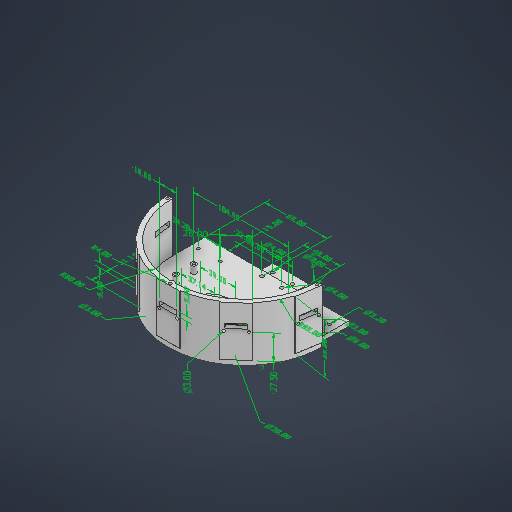
# Autodesk Inventor part: Mitad_1
Saved by Autodesk Inventor 2026.2 (Build 302298000, 298)
## iProperties
Created: 2025-10-28
Part Number: Mitad_1
Material: Genérico
Document SubType Name: Modeling
Designer: 100094631
Density: 1 g/cm^3
Appearance: Valor por defecto
Author: 100094631
## iProperties of the stored document Mitad_1_3DPrint.ipt
Created: 2026-02-23
Part Number: Mitad_1_3DPrint
Material: Genérico
Document SubType Name: Modeling
Designer: yahir
Density: 1 g/cm^3
Appearance: Valor por defecto
Author: yahir
Autodesk Inventor part; units mm, degrees
ref_plane "YZ Plane" through (0, 0, 0) normal (1, 0, 0) x (0, 1, 0)
ref_plane "XZ Plane" through (0, 0, 0) normal (0, 1, 0) x (-1, 0, 0)
ref_plane "XY Plane" through (0, 0, 0) normal (0, 0, 1) x (1, 0, 0)
sketch "Boceto2" plane through (0, 0, 0) normal (0, 1, 0) x (-1, 0, 0)
  arc A0 (85, 0) -> (-85, 0) centre (0, 0) ccw
  line L0 (85, 0) -> (80, 0)
  line L1 (-80, 0) -> (-85, 0)
  line L2 (80, 0) -> (80, -36)
  line L3 (-80, 0) -> (-80, -36)
  line L4 (-80, -36) -> (80, -36)
  point P0 (0, 0)
  point P1 (0, 85)
  dimension "d228" = 85
  dimension "d229" = 5
  dimension "d461" = 36
  dimension "d462" = 36
  constraints: 10 end point, 3 point on circle, 2 vertical, 1 centre point, 1 horizontal, 1 point on line
  measures "d228" distance of point (0, 0) L1.end
  measures "d229" distance of L0.start L0.end
  measures "d461" distance of L0.end L2.end
  measures "d462" distance of L1.start L3.end
extrude "Extrusión1" add sketch "Boceto2" along normal blind 5
sketch "Boceto6" plane through (0, 5, 0) normal (0, 1, 0) x (1, 0, 0)
  circle A0 centre (48.25, 21) radius 1.6
  circle A1 centre (72.45, 21) radius 1.6
  circle A2 centre (-72.45, 21) radius 1.6
  line L0 (80, 36) -> (-80, 36) projected
  line L1 (80, 36) -> (80, 21)
  line L2 (80, 0) -> (80, 36) projected
  line L3 (80, 21) -> (72.45, 21)
  line L4 (-80, 36) -> (-80, 0) projected
  line L5 (-80, 36) -> (-80, 21)
  line L6 (-80, 21) -> (-72.45, 21)
  line L7 (72.45, 21) -> (48.25, 21)
  line L8 (-72.45, 21) -> (-48.25, 21)
  circle A3 centre (-48.25, 21) radius 1.6
  dimension "d59" = 3.2
  dimension "d60" = 3.2
  dimension "d63" = 3.2
  dimension "d468" = 15
  dimension "d469" = 7.55
  dimension "d471" = 15
  dimension "d472" = 7.55
  dimension "d502" = 24.2
  dimension "d503" = 24.2
  dimension "d504" = 3.2
  constraints: 12 end point, 4 centre point, 3 point on line, 2 perpendicular, 1 coincident, 1 horizontal
  measures "d59" diameter of A0
  measures "d60" diameter of A1
  measures "d63" diameter of A2
  measures "d468" distance of L0.start L1.end
  measures "d469" distance of L1.end L3.end
  measures "d471" distance of L0.end L5.end
  measures "d472" distance of L5.end L6.end
  measures "d502" distance of L3.end L7.end
  measures "d503" distance of L6.end L8.end
  measures "d504" diameter of A3
extrude "Extrusión4" cut sketch "Boceto6" against normal blind 5
sketch "Boceto7" plane through (0, 5, 0) normal (0, 1, 0) x (1, 0, 0)
  line L0 (0, 0) -> (0, -85)
  line L1 (0, 0) -> (55.2031, -64.6345)
  line L2 (0, 0) -> (83.9535, -13.2969)
  arc A0 (-80, 0) -> (80, 0) centre (0, 0) ccw
  line L3 (-85, 0) -> (-80, 0)
  line L4 (80, 0) -> (85, 0)
  line L5 (0, -85) -> (13, -85)
  arc A1 (-85, 0) -> (85, 0) centre (0, 0) ccw projected
  line L6 (0, -85) -> (-13, -85)
  line L7 (-13, -85) -> (-13, -84)
  line L8 (13, -85) -> (13, -84)
  line L9 (0, 0) -> (-55.2031, -64.6345)
  line L10 (0, 0) -> (85, 0) construction
  line L11 (0, 0) -> (85, 0) construction
  line L12 (0, 0) -> (-83.9535, -13.2969)
  line L13 (0, 0) -> (90.9011, 0) construction
  line L14 (0, 0) -> (55.2031, -64.6345)
  line L15 (55.2031, -64.6345) -> (65.0884, -56.1917)
  line L16 (55.2031, -64.6345) -> (45.3178, -73.0773)
  line L17 (45.3178, -73.0773) -> (44.6684, -72.3169)
  line L18 (65.0884, -56.1917) -> (64.4389, -55.4313)
  line L19 (0, 0) -> (83.9535, -13.2969)
  line L20 (83.9535, -13.2969) -> (85.9872, -0.457)
  line L21 (83.9535, -13.2969) -> (81.9199, -26.1369)
  line L22 (81.9199, -26.1369) -> (80.9322, -25.9804)
  line L23 (85.9872, -0.457) -> (84.9995, -0.3005)
  line L24 (0, 0) -> (-55.2031, -64.6345)
  line L25 (-55.2031, -64.6345) -> (-45.3178, -73.0773)
  line L26 (-55.2031, -64.6345) -> (-65.0884, -56.1917)
  line L27 (-65.0884, -56.1917) -> (-64.4389, -55.4313)
  line L28 (-45.3178, -73.0773) -> (-44.6684, -72.3169)
  line L29 (0, 0) -> (-83.9535, -13.2969)
  line L30 (-83.9535, -13.2969) -> (-81.9199, -26.1369)
  line L31 (-83.9535, -13.2969) -> (-85.9872, -0.457)
  line L32 (-85.9872, -0.457) -> (-84.9995, -0.3005)
  line L33 (-81.9199, -26.1369) -> (-80.9322, -25.9804)
  arc A2 (-85, 0) -> (-84.9995, -0.3005) centre (0, 0) ccw
  arc A3 (-80.9322, -25.9804) -> (-64.4389, -55.4313) centre (0, 0) ccw
  arc A4 (-44.6684, -72.3169) -> (-13, -84) centre (0, 0) ccw
  arc A5 (13, -84) -> (44.6684, -72.3169) centre (0, 0) ccw
  arc A6 (64.4389, -55.4313) -> (80.9322, -25.9804) centre (0, 0) ccw
  arc A7 (84.9995, -0.3005) -> (85, 0) centre (0, 0) ccw
  point P0 (0, 0)
  point P1 (-80, 0)
  dimension "d234" = 40.5
  dimension "d235" = 81
  dimension "d237" = 13
  dimension "d238" = 13
  dimension "d241" = 171
  dimension "d242" = 13
  dimension "d243" = 13
  dimension "d244" = 13
  dimension "d245" = 13
  dimension "d246" = 13
  dimension "d247" = 13
  dimension "d248" = 13
  dimension "d249" = 13
  constraints: 68 end point, 17 point on circle, 7 centre point, 7 horizontal, 5 perpendicular, 3 tangent, 2 vertical, 1 coincident, 1 equal length
  measures "d234" angle of L1 L0
  measures "d235" angle of L2 L0
  measures "d237" distance of L0.end L5.end
  measures "d238" distance of L0.end L6.end
  measures "d241" angle of L12 L13
  measures "d242" distance of L15.start L15.end
  measures "d243" distance of L15.start L16.end
  measures "d244" distance of L21.start L20.end
  measures "d245" distance of L21.start L21.end
  measures "d246" distance of L24.end L25.end
  measures "d247" distance of L24.end L27.start
  measures "d248" distance of L29.end L33.start
  measures "d249" distance of L29.end L31.end
extrude "Extrusión5" add sketch "Boceto7" along normal blind 55 contours A0 L1 A1 L0 | L0 A1 L9 A0 | A0 L2 A1 L1 | A0 L4 A1 L2 | L9 A1 L12 A0 | L12 A1 L3 A0 | A1 L8 L5 | L6 L7 A1 | L16 L17 A1 | A1 L18 L15 | L21 L22 A1 | A1 L23 L20 | L26 L27 A1 | A1 L28 L25 | L31 L32 A1 | A1 L33 L30
sketch "Boceto22" plane through (0, 5, 0) normal (0, 1, 0) x (1, 0, 0)
  ellipse E0 centre (0, -30) end of major axis (0, -12.5) minor radius 25
  line L0 (0, -30) -> (-0.3651, -30)
  line L1 (-80, 36) -> (0, 36)
  line L2 (80, 36) -> (-80, 36) projected
  line L3 (-80, 36) -> (-80, 0) projected
  line L4 (-80, 36) -> (0, 36)
  line L5 (0, 36) -> (0, -30)
  point P0 (0, 0)
  dimension "d473" = 80
  constraints: 8 end point, 1 collinear, 1 horizontal, 1 midpoint, 1 vertical, 2 other
  measures "d473" distance of L1.start L1.end
extrude "Extrusión15" add sketch "Boceto22" along normal blind 3.3
sketch "Boceto25" plane through (0, 60, 0) normal (0, 1, 0) x (1, 0, 0)
  circle A0 centre (82.75, -3) radius 1.5
  circle A1 centre (-82.75, -3) radius 1.5
  circle A2 centre (0, -82.5) radius 1.5
  line L0 (0, -85) -> (0, -82.5)
  line L1 (82.75, 0) -> (82.75, -3)
  line L2 (-82.75, 0) -> (-82.75, -3)
  line L3 (85, 0) -> (80, 0) projected
  line L4 (80, 0) -> (82.75, 0)
  line L5 (-80, 0) -> (-82.75, 0)
  line L6 (-80, 0) -> (-85, 0) projected
  arc A3 (4, -82.5) -> (-4, -82.5) centre (0, -82.5) ccw
  line L7 (0, -82.5) -> (-4, -82.5)
  line L8 (0, -82.5) -> (4, -82.5)
  point P0 (0, 0)
  point P1 (-1.5, -82.5)
  point P2 (1.5, -82.5)
  dimension "d200" = 3
  dimension "d203" = 3
  dimension "d205" = 3
  dimension "d264" = 3
  dimension "d267" = 3
  dimension "d423" = 2.75
  dimension "d424" = 2.75
  dimension "d460" = 2.5
  constraints: 14 end point, 4 centre point, 3 point on line, 2 point on circle, 1 coincident, 1 horizontal, 1 vertical
  measures "d200" diameter of A0
  measures "d203" diameter of A1
  measures "d205" diameter of A2
  measures "d264" distance of L1.start L1.end
  measures "d267" distance of L2.start L2.end
  measures "d423" distance of L3.end L4.end
  measures "d424" distance of L5.start L5.end
  measures "d460" distance of L0.start L0.end
extrude "Extrusión17" cut sketch "Boceto25" against normal blind 5 contours A0 | A1 | L8 L7 A2 | A2 L0 L8 | L7 L0 A2
sketch "Boceto27" plane through (0, 8.3, 0) normal (0, 1, 0) x (1, 0, 0)
  ellipse E0 centre (0, -30) end of major axis (-25, -30) minor radius 17.5 projected
  circle A0 centre (0, -30) radius 15
  line L0 (0, -30) -> (-19.5, -30)
  line L1 (0, -30) -> (19.5, -30)
  circle A1 centre (19.5, -30) radius 2
  circle A2 centre (-19.5, -30) radius 2
  point P0 (0, 0)
  dimension "d252" = 30
  dimension "d253" = 19.5
  dimension "d254" = 19.5
  dimension "d255" = 4
  dimension "d256" = 4
  constraints: 4 end point, 3 centre point, 3 coincident, 2 horizontal, 1 other
  measures "d252" diameter of A0
  measures "d253" distance of L0.start L0.end
  measures "d254" distance of L0.start L1.end
  measures "d255" diameter of A1
  measures "d256" diameter of A2
extrude "Extrusión19" cut sketch "Boceto27" against normal blind 15 contours L1 L0 A0 | A2 | A0 L0 L1 | A1
sketch "Boceto31" plane through (-13, 5, 85) normal (0, 0, 1) x (1, 0, 0)
  line L0 (26, 0) -> (26, 55) projected
  line L1 (26, 0) -> (13, 0)
  line L2 (-12, 0) -> (38, 0) projected
  line L3 (13, 0) -> (13, 27.5)
  line L4 (13, 27.5) -> (23, 27.5)
  line L5 (13, 27.5) -> (3, 27.5)
  circle A0 centre (3, 27.5) radius 1.5
  circle A1 centre (23, 27.5) radius 1.5
  point P0 (13, -5)
  dimension "d282" = 13
  dimension "d283" = 27.5
  dimension "d285" = 10
  dimension "d286" = 3
  dimension "d287" = 3
  constraints: 8 end point, 2 centre point, 2 coincident, 2 horizontal, 1 midpoint, 1 perpendicular
  measures "d282" distance of L0.start L1.end
  measures "d283" distance of L1.end L3.end
  measures "d285" distance of L3.end L5.end
  measures "d286" diameter of A0
  measures "d287" diameter of A1
extrude "Extrusión23" cut sketch "Boceto31" against normal blind 3
sketch "Boceto32" plane through (65.0884, 5, 56.1917) normal (0.6494, 0, 0.7604) x (0.7604, 0, -0.6494)
  line L0 (-26, 0) -> (-26, 55) projected
  line L1 (-26, 0) -> (-13, 0)
  line L2 (-54.632, 0) -> (-10.3349, 0) projected
  line L3 (-13, 0) -> (-13, 27.5)
  line L4 (-13, 27.5) -> (-3, 27.5)
  line L5 (-13, 27.5) -> (-23, 27.5)
  circle A0 centre (-23, 27.5) radius 1.5
  circle A1 centre (-3, 27.5) radius 1.5
  point P0 (-13, -5)
  dimension "d290" = 13
  dimension "d291" = 27.5
  dimension "d292" = 10
  dimension "d293" = 10
  dimension "d294" = 3
  dimension "d295" = 3
  constraints: 8 end point, 2 centre point, 2 coincident, 2 horizontal, 1 perpendicular, 1 point on line
  measures "d290" distance of L0.start L1.end
  measures "d291" distance of L1.end L3.end
  measures "d292" distance of L3.end L4.end
  measures "d293" distance of L3.end L5.end
  measures "d294" diameter of A0
  measures "d295" diameter of A1
extrude "Extrusión24" cut sketch "Boceto32" against normal blind 3
sketch "Boceto33" plane through (85.9872, 5, 0.457) normal (0.9877, 0, 0.1564) x (0.1564, 0, -0.9877)
  line L0 (0.0086, 0) -> (-12.9914, 0)
  line L1 (-0.4852, 0) -> (-93, 0) projected
  line L2 (-12.9914, 0) -> (-12.9914, 27.5)
  line L3 (-12.9914, 27.5) -> (-2.9914, 27.5)
  line L4 (-12.9914, 27.5) -> (-22.9914, 27.5)
  circle A0 centre (-22.9914, 27.5) radius 1.5
  circle A1 centre (-2.9914, 27.5) radius 1.5
  point P0 (-13, -5)
  point P1 (-25.5148, 0)
  dimension "d298" = 13
  dimension "d299" = 27.5
  dimension "d300" = 10
  dimension "d301" = 10
  dimension "d302" = 3
  dimension "d303" = 3
  constraints: 8 end point, 2 centre point, 2 coincident, 2 perpendicular, 1 horizontal, 1 point on line
  measures "d298" distance of L0.start L0.end
  measures "d299" distance of L0.end L2.end
  measures "d300" distance of L2.end L3.end
  measures "d301" distance of L2.end L4.end
  measures "d302" diameter of A0
  measures "d303" diameter of A1
extrude "Extrusión25" cut sketch "Boceto33" against normal blind 3
sketch "Boceto34" plane through (-45.3178, 5, 73.0773) normal (-0.6494, 0, 0.7604) x (0.7604, 0, 0.6494)
  line L0 (67, 0) -> (-73.8325, 0) projected
  line L1 (-26.0047, 0) -> (-13.0047, 0)
  line L2 (-13.0047, 0) -> (-13.0047, 27.5)
  line L3 (-15.6651, 0) -> (28.632, 0) projected
  line L4 (-13.0047, 0) -> (14.4953, 0) construction
  line L5 (-13.0047, 27.5) -> (-3.0047, 27.5)
  line L6 (-13.0047, 27.5) -> (-23.0047, 27.5)
  circle A0 centre (-23.0047, 27.5) radius 1.5
  circle A1 centre (-3.0047, 27.5) radius 1.5
  point P0 (-13, -5)
  point P1 (47.8325, 0)
  dimension "d306" = 13
  dimension "d307" = 27.5
  dimension "d308" = 90
  dimension "d309" = 10
  dimension "d310" = 10
  dimension "d311" = 3
  dimension "d312" = 3
  constraints: 10 end point, 3 horizontal, 2 centre point, 2 coincident, 2 perpendicular, 2 point on line
  measures "d306" distance of L1.start L1.end
  measures "d307" distance of L1.end L2.end
  measures "d308" angle of L4 L2
  measures "d309" distance of L2.end L5.end
  measures "d310" distance of L2.end L6.end
  measures "d311" diameter of A0
  measures "d312" diameter of A1
extrude "Extrusión26" cut sketch "Boceto34" against normal blind 3
sketch "Boceto35" plane through (-81.9199, 5, 26.1369) normal (-0.9877, 0, 0.1564) x (0.1564, 0, 0.9877)
  line L0 (-27.7935, 0) -> (-24.5935, 0) projected
  line L1 (-25.9863, 0) -> (-12.9863, 0)
  line L2 (-12.9863, 0) -> (-12.9863, 27.5)
  line L3 (-12.9863, 27.5) -> (-2.9863, 27.5)
  line L4 (-12.9863, 27.5) -> (-22.9863, 27.5)
  circle A0 centre (-22.9863, 27.5) radius 1.5
  circle A1 centre (-2.9863, 27.5) radius 1.5
  point P0 (-13, -5)
  dimension "d315" = 13
  dimension "d316" = 27.5
  dimension "d317" = 10
  dimension "d318" = 10
  dimension "d319" = 3
  dimension "d320" = 3
  constraints: 8 end point, 2 centre point, 2 coincident, 2 perpendicular, 1 collinear, 1 horizontal, 1 point on line
  measures "d315" distance of L1.start L1.end
  measures "d316" distance of L1.end L2.end
  measures "d317" distance of L2.end L3.end
  measures "d318" distance of L2.end L4.end
  measures "d319" diameter of A0
  measures "d320" diameter of A1
extrude "Extrusión27" cut sketch "Boceto35" against normal blind 3
sketch "Boceto36" plane through (-13, 5, 85) normal (0, 0, 1) x (1, 0, 0)
  circle A0 centre (3, 27.5) radius 1.5 projected
  line L0 (3, 27.5) -> (13, 27.5)
  line L1 (13, 27.5) -> (13, 32.5)
  line L2 (4, 32.5) -> (4, 35)
  line L3 (4, 35) -> (22, 35)
  line L4 (22, 35) -> (22, 30)
  line L5 (22, 30) -> (4, 30)
  line L6 (4, 30) -> (4, 32.5)
  point P0 (13, -5)
  dimension "d336" = 10
  dimension "d337" = 5
  dimension "d340" = 2.5
  dimension "d358" = 18
  dimension "d359" = 5
  dimension "d360" = 18
  constraints: 14 end point, 2 horizontal, 2 perpendicular, 2 vertical
  measures "d336" distance of L0.start L0.end
  measures "d337" distance of L0.end L1.end
  measures "d340" distance of L2.start L2.end
  measures "d358" distance of L2.end L3.end
  measures "d359" distance of L3.end L4.end
  measures "d360" distance of L4.end L5.end
extrude "Extrusión28" cut sketch "Boceto36" against normal blind 6 contours L5 L6 L2 L3 L4
sketch "Boceto37" plane through (65.0884, 5, 56.1917) normal (0.6494, 0, 0.7604) x (0.7604, 0, -0.6494)
  circle A0 centre (-23, 27.5) radius 1.5 projected
  line L0 (-23, 27.5) -> (-13, 27.5)
  line L1 (-13, 27.5) -> (-13, 32.5)
  line L2 (-13, 32.5) -> (-4, 32.5)
  line L3 (-4, 32.5) -> (-4, 30)
  line L4 (-4, 30) -> (-22, 30)
  line L5 (-22, 30) -> (-22, 35)
  line L6 (-22, 35) -> (-4, 35)
  line L7 (-4, 35) -> (-4, 32.5)
  point P0 (-13, -5)
  dimension "d348" = 10
  dimension "d349" = 5
  dimension "d350" = 9
  dimension "d351" = 2.5
  dimension "d352" = 18
  dimension "d354" = 5
  dimension "d355" = 18
  constraints: 16 end point, 3 vertical, 2 horizontal, 2 perpendicular
  measures "d348" distance of L0.start L0.end
  measures "d349" distance of L0.end L1.end
  measures "d350" distance of L1.end L2.end
  measures "d351" distance of L2.end L3.end
  measures "d352" distance of L3.end L4.end
  measures "d354" distance of L4.end L5.end
  measures "d355" distance of L5.end L6.end
extrude "Extrusión29" cut sketch "Boceto37" against normal blind 6 contours L4 L5 L6 L7 L2 L1 | L1 L2 L3 L4
sketch "Boceto38" plane through (85.9872, 5, 0.457) normal (0.9877, 0, 0.1564) x (0.1564, 0, -0.9877)
  circle A0 centre (-22.9914, 27.5) radius 1.5 projected
  line L0 (-22.9914, 27.5) -> (-12.9914, 27.5)
  line L1 (-12.9914, 27.5) -> (-12.9914, 32.5)
  line L2 (-12.9914, 32.5) -> (-3.9914, 32.5)
  line L3 (-3.9914, 35) -> (-21.9914, 35)
  line L4 (-21.9914, 35) -> (-21.9914, 30)
  line L5 (-21.9914, 30) -> (-3.9914, 30)
  line L6 (-3.9914, 30) -> (-3.9914, 35)
  point P0 (-13, -5)
  dimension "d361" = 10
  dimension "d362" = 5
  dimension "d364" = 2.5
  dimension "d366" = 5
  dimension "d367" = 18
  constraints: 14 end point, 3 horizontal, 3 perpendicular, 1 vertical
  measures "d361" distance of L0.start L0.end
  measures "d362" distance of L0.end L1.end
  measures "d364" distance of L2.end L3.start
  measures "d366" distance of L3.end L4.end
  measures "d367" distance of L4.end L5.end
extrude "Extrusión30" cut sketch "Boceto38" against normal blind 6 contours L5 L4 L3 L6 L2 L1 | L1 L2 L6 L5
sketch "Boceto40" plane through (-45.3178, 5, 73.0773) normal (-0.6494, 0, 0.7604) x (0.7604, 0, 0.6494)
  circle A0 centre (-23.0047, 27.5) radius 1.5 projected
  line L0 (-23.0047, 27.5) -> (-13.0047, 27.5)
  line L1 (-13.0047, 27.5) -> (-13.0047, 32.5)
  line L2 (-13.0047, 32.5) -> (-4.0047, 32.5)
  line L3 (-4.0047, 32.5) -> (-4.0047, 35)
  line L4 (-4.0047, 35) -> (-22.0047, 35)
  line L5 (-22.0047, 35) -> (-22.0047, 30)
  line L6 (-22.0047, 30) -> (-4.0047, 30)
  line L7 (-4.0047, 30) -> (-4.0047, 32.5)
  point P0 (-13, -5)
  dimension "d370" = 10
  dimension "d371" = 5
  dimension "d372" = 9
  dimension "d373" = 2.5
  dimension "d374" = 18
  dimension "d375" = 5
  dimension "d376" = 18
  constraints: 16 end point, 4 perpendicular, 3 horizontal
  measures "d370" distance of L0.start L0.end
  measures "d371" distance of L0.end L1.end
  measures "d372" distance of L1.end L2.end
  measures "d373" distance of L2.end L3.end
  measures "d374" distance of L3.end L4.end
  measures "d375" distance of L4.end L5.end
  measures "d376" distance of L5.end L6.end
extrude "Extrusión31" cut sketch "Boceto40" against normal blind 6 contours L6 L5 L4 L3 L2 L1 | L1 L2 L7 L6
sketch "Boceto41" plane through (-81.9199, 5, 26.1369) normal (-0.9877, 0, 0.1564) x (0.1564, 0, 0.9877)
  circle A0 centre (-22.9863, 27.5) radius 1.5 projected
  line L0 (-22.9863, 27.5) -> (-12.9863, 27.5)
  line L1 (-12.9863, 27.5) -> (-12.9863, 32.5)
  line L2 (-12.9863, 32.5) -> (-3.9863, 32.5)
  line L3 (-3.9863, 35) -> (-21.9863, 35)
  line L4 (-21.9863, 35) -> (-21.9863, 30)
  line L5 (-21.9863, 30) -> (-3.9863, 30)
  line L6 (-3.9863, 30) -> (-3.9863, 35)
  point P0 (-13, -5)
  dimension "d379" = 10
  dimension "d380" = 5
  dimension "d382" = 2.5
  dimension "d384" = 5
  dimension "d385" = 18
  constraints: 14 end point, 3 horizontal, 3 perpendicular, 1 vertical
  measures "d379" distance of L0.start L0.end
  measures "d380" distance of L0.end L1.end
  measures "d382" distance of L2.end L3.start
  measures "d384" distance of L3.end L4.end
  measures "d385" distance of L4.end L5.end
extrude "Extrusión32" cut sketch "Boceto41" against normal blind 6 contours L5 L4 L3 L6 L2 L1 | L1 L2 L6 L5
sketch "Boceto42" plane through (0, 5, 0) normal (0, 1, 0) x (1, 0, 0)
  circle A0 centre (-72.45, 21) radius 1.6 projected
  circle A1 centre (72.45, 21) radius 1.6 projected
  circle A2 centre (-19.5, -30) radius 2 projected
  circle A3 centre (-52.45, -4) radius 3
  circle A4 centre (-52.45, -24) radius 3
  circle A5 centre (52.45, -24) radius 3
  circle A6 centre (52.45, -4) radius 3
  line L0 (-52.45, -4) -> (-52.45, -24)
  line L1 (52.45, -4) -> (52.45, -24)
  line L2 (-72.45, 21) -> (-72.45, -4)
  line L3 (-72.45, -4) -> (-52.45, -4)
  line L4 (72.45, 21) -> (72.45, -4)
  line L5 (72.45, -4) -> (52.45, -4)
  point P0 (0, 0)
  dimension "d437" = 6
  dimension "d446" = 20
  dimension "d533" = 20
  dimension "d537" = 25
  dimension "d538" = 20
  dimension "d539" = 25
  dimension "d540" = 20
  constraints: 12 end point, 4 centre point, 4 vertical, 2 perpendicular
  measures "d437" diameter of A4
  measures "d446" distance of L0.start L0.end
  measures "d533" distance of L1.start L1.end
  measures "d537" distance of L2.start L2.end
  measures "d538" distance of L2.end L3.end
  measures "d539" distance of L4.start L4.end
  measures "d540" distance of L4.end L1.start
extrude "Extrusión33" add sketch "Boceto42" along normal blind 8 contours A4 | A3 L0 L3 | L3 L0 A3 | A5 | A6 L1 L5 | L5 L1 A6
sketch "Boceto43" plane through (-72.45, 13, -5) normal (0, 1, 0) x (1, 0, 0)
  circle A0 centre (20, -9) radius 3 projected
  circle A1 centre (20, -9) radius 1.5
  circle A2 centre (20, -29) radius 3 projected
  circle A3 centre (20, -29) radius 1.5
  circle A4 centre (124.9, -29) radius 3 projected
  circle A5 centre (124.9, -29) radius 1.5
  circle A6 centre (124.9, -9) radius 3 projected
  circle A7 centre (124.9, -9) radius 1.5
  point P0 (72.45, -5)
  dimension "d440" = 3
  dimension "d441" = 3
  dimension "d442" = 3
  dimension "d443" = 3
  constraints: 4 centre point, 4 coincident
  measures "d440" diameter of A1
  measures "d441" diameter of A3
  measures "d442" diameter of A5
  measures "d443" diameter of A7
extrude "Extrusión34" cut sketch "Boceto43" against normal blind 4 contours A1 | A3 | A5 | A7
extrude "Extrusión35" add sketch "Boceto25" against normal blind 5 contours A2 L7 A3 L8
sketch "Boceto46" plane through (80, 0, -36) normal (0, 0, -1) x (-1, 0, 0)
  line L0 (95, 0) -> (65, 0) projected
  line L1 (80, 0) -> (60, 0)
  line L2 (60, 0) -> (60, 2.5)
  line L3 (60, 2.5) -> (100, 2.5)
  line L4 (100, 2.5) -> (100, 0)
  line L5 (100, 0) -> (80, 0)
  dimension "d478" = 20
  dimension "d479" = 2.5
  dimension "d480" = 40
  dimension "d481" = 2.5
  constraints: 10 end point, 2 perpendicular, 2 point on line, 1 collinear
  measures "d478" distance of L1.start L1.end
  measures "d479" distance of L1.end L2.end
  measures "d480" distance of L2.end L3.end
  measures "d481" distance of L3.end L4.end
extrude "Extrusión36" add sketch "Boceto46" along normal blind 15
sketch "Boceto48" plane through (-20, 2.5, -36) normal (0, 1, 0) x (1, 0, 0)
  line L0 (40, 0) -> (0, 0) projected
  line L1 (20, 0) -> (20, 6)
  line L2 (20, 6) -> (9, 6)
  line L3 (20, 6) -> (31, 6)
  circle A0 centre (9, 6) radius 2
  circle A1 centre (31, 6) radius 2
  line L4 (20, 0) -> (20, -6)
  line L5 (20, -6) -> (9, -6)
  line L6 (20, -6) -> (31, -6)
  circle A2 centre (9, -6) radius 2
  circle A3 centre (31, -6) radius 2
  point P0 (20, -36)
  dimension "d488" = 6
  dimension "d489" = 11
  dimension "d490" = 11
  dimension "d491" = 4
  dimension "d492" = 4
  dimension "d495" = 6
  dimension "d496" = 11
  dimension "d497" = 11
  dimension "d498" = 4
  dimension "d499" = 4
  constraints: 12 end point, 4 centre point, 4 coincident, 2 horizontal, 2 perpendicular, 2 vertical, 1 midpoint
  measures "d488" distance of L1.start L1.end
  measures "d489" distance of L1.end L2.end
  measures "d490" distance of L1.end L3.end
  measures "d491" diameter of A0
  measures "d492" diameter of A1
  measures "d495" distance of L1.start L4.end
  measures "d496" distance of L4.end L5.end
  measures "d497" distance of L4.end L6.end
  measures "d498" diameter of A2
  measures "d499" diameter of A3
extrude "Extrusión38" cut sketch "Boceto48" against normal blind 2.5 contours A0 | A1
extrude "Extrusión39" cut sketch "Boceto48" along normal mid plane 7 contours A3 | A2
sketch "Boceto49" plane through (0, 5, 0) normal (0, 1, 0) x (1, 0, 0)
  line L0 (-21.57, -51.7456) -> (21.57, -51.7456)
  line L1 (21.57, -51.7456) -> (21.57, -72.8856)
  line L2 (21.57, -72.8856) -> (-21.57, -72.8856)
  line L3 (-21.57, -72.8856) -> (-21.57, -51.7456)
  line L4 (21.57, -51.7456) -> (21.57, -62.3156)
  line L5 (21.57, -51.7456) -> (-21.57, -51.7456)
  point P0 (0, 0)
  constraints: 12 end point, 2 parallel, 1 horizontal, 1 midpoint, 1 perpendicular
extrude "Extrusión40" add sketch "Boceto49" along normal blind 5
sketch "Boceto50" plane through (0, 10, 0) normal (0, 1, 0) x (1, 0, 0)
  line L0 (21.57, -72.8856) -> (15.07, -72.8856)
  line L1 (-21.57, -72.8856) -> (21.57, -72.8856) projected
  line L2 (15.07, -72.8856) -> (15.07, -70.3856)
  line L3 (-21.57, -51.7456) -> (-21.57, -72.8856) projected
  line L4 (-21.57, -51.7456) -> (-15.07, -51.7456)
  line L5 (21.57, -51.7456) -> (-21.57, -51.7456) projected
  line L6 (-15.07, -51.7456) -> (-15.07, -54.2456)
  circle A0 centre (15.07, -70.3856) radius 1.5
  circle A1 centre (-15.07, -54.2456) radius 1.5
  point P0 (0, 0)
  dimension "d519" = 6.5
  dimension "d520" = 2.5
  dimension "d521" = 6.5
  dimension "d522" = 2.5
  dimension "d523" = 3
  dimension "d524" = 3
  constraints: 8 end point, 2 centre point, 2 coincident, 2 point on line, 1 perpendicular, 1 vertical
  measures "d519" distance of L0.start L0.end
  measures "d520" distance of L0.end L2.end
  measures "d521" distance of L3.start L4.end
  measures "d522" distance of L4.end L6.end
  measures "d523" diameter of A0
  measures "d524" diameter of A1
extrude "Extrusión42" cut sketch "Boceto50" against normal blind 5
sketch "Boceto51" plane through (0, 10, 0) normal (0, 1, 0) x (1, 0, 0)
  line L0 (-21.57, -51.7456) -> (-21.57, -72.8856) projected
  line L1 (-21.57, -51.7456) -> (-18.57, -51.7456)
  line L2 (21.57, -51.7456) -> (-21.57, -51.7456) projected
  line L3 (-18.57, -51.7456) -> (-18.57, -72.8856)
  line L4 (-21.57, -72.8856) -> (21.57, -72.8856) projected
  line L5 (-21.57, -72.8856) -> (-21.57, -51.7456)
  line L6 (21.57, -72.8856) -> (21.57, -51.7456) projected
  line L7 (21.57, -72.8856) -> (18.57, -72.8856)
  line L8 (18.57, -72.8856) -> (18.57, -51.7456)
  line L9 (18.57, -51.7456) -> (21.57, -51.7456)
  line L10 (21.57, -51.7456) -> (21.57, -72.8856)
  point P0 (0, 0)
  dimension "d527" = 3
  dimension "d528" = 3
  constraints: 14 end point, 4 perpendicular, 3 point on line, 1 horizontal, 1 parallel
  measures "d527" distance of L0.start L1.end
  measures "d528" distance of L4.end L7.end
extrude "Extrusión43" cut sketch "Boceto51" against normal blind 5 contours L1 L3 L4 L0 | L2 L6 L4 L8
